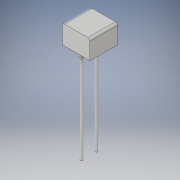
# Autodesk Inventor part: Capacitor
Saved by Autodesk Inventor 2019 (Build 230136000, 136)
## iProperties
Created: 2020-04-10
Part Number: Capacitor
Material: Generic
Document SubType Name: Modeling
Designer: darkl
Density: 1 g/cm^3
Appearance: Default
Author: darkl
Autodesk Inventor part; units mm, degrees
ref_plane "YZ Plane" through (0, 0, 0) normal (1, 0, 0) x (0, 1, 0)
ref_plane "XZ Plane" through (0, 0, 0) normal (0, 1, 0) x (-1, 0, 0)
ref_plane "XY Plane" through (0, 0, 0) normal (0, 0, 1) x (1, 0, 0)
sketch "Sketch3" plane through (0, 0, 0) normal (0, 1, 0) x (-1, 0, 0)
  line L0 (2.9769, -4.8208) -> (-3.5231, -4.8208)
  line L1 (-3.5231, -4.8208) -> (-3.5231, -11.3208)
  line L2 (-3.5231, -11.3208) -> (2.9769, -11.3208)
  line L3 (2.9769, -11.3208) -> (2.9769, -4.8208)
  point P0 (0, 0)
  dimension "d0" = 6.5
  dimension "d1" = 6.5
  constraints: 8 end point, 2 parallel, 1 horizontal, 1 perpendicular
  measures "d0" distance of L2.end L1.end
  measures "d1" distance of L2.end L0.start
extrude "Extrusion1" add sketch "Sketch3" along normal blind 4.5
fillet "Fillet1" radius 0.5 1 edges at (3.5231, 4.5, -8.0708)
fillet "Fillet2" radius 0.5 1 edges at (-2.9769, 4.5, -8.0708)
sketch "Sketch5" plane through (0, 0, 0) normal (0, -1, 0) x (1, 0, 0)
  circle A0 centre (0, -9.8613) radius 0.5
  circle A1 centre (0, -6.3617) radius 0.5
  point P0 (0, 0)
  dimension "d6" = 1
  dimension "d8" = 1
  constraints: 2 centre point
  measures "d6" diameter of A0
  measures "d8" diameter of A1
extrude "Extrusion2" add sketch "Sketch5" along normal blind 2 contours A0
sketch "Sketch7" plane through (0, 0, 0) normal (0, -1, 0) x (1, 0, 0)
  circle A0 centre (0, -9.8613) radius 0.5
  circle A1 centre (0, -6.3617) radius 0.5
  point P0 (0, 0)
  point P1 (0, 0)
  dimension "d15" = 1
  dimension "d16" = 1
  constraints: 2 centre point
  measures "d15" diameter of A0
  measures "d16" diameter of A1
extrude "Extrusion4" add sketch "Sketch7" along normal blind 2 contours A1
sketch "Sketch8" plane through (0, -2, -6.3617) normal (0, -1, 0) x (1, 0, 0)
  circle A0 centre (0, 0) radius 0.3
  point P0 (0, 6.3617)
  dimension "d19" = 0.6
  constraints: 1 centre point
  measures "d19" diameter of A0
extrude "Extrusion5" add sketch "Sketch8" along normal blind 21
sketch "Sketch9" plane through (0, -2, -9.8613) normal (0, -1, 0) x (1, 0, 0)
  circle A0 centre (0, 0) radius 0.3
  point P0 (0, 9.8613)
  dimension "d22" = 0.6
  constraints: 1 centre point
  measures "d22" diameter of A0
extrude "Extrusion6" add sketch "Sketch9" along normal blind 21
fillet "Fillet3" radius 0.5 1 edges at (-0.5, -2, -6.3617)
fillet "Fillet4" radius 0.5 1 edges at (-0.5, -2, -9.8613)
fillet "Fillet5" radius 0.2 1 edges at (-0.3, -23, -6.3617)
fillet "Fillet6" radius 0.2 1 edges at (-0.3, -23, -9.8613)
body "Solid1"
